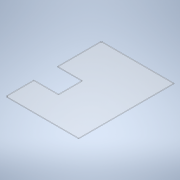
# Autodesk Inventor part: MountingWallSide2
Saved by Autodesk Inventor 2020 (Build 240168000, 168)
## iProperties
Created: 2020-04-26
Part Number: MountingWallSide2
Material: Типовые
Document SubType Name: Modeling
Designer: Михаил
Density: 1 g/cm^3
Appearance: По умолчанию
Author: Михаил
Autodesk Inventor part; units mm, degrees
ref_plane "YZ Plane" through (0, 0, 0) normal (1, 0, 0) x (0, 1, 0)
ref_plane "XZ Plane" through (0, 0, 0) normal (0, 1, 0) x (-1, 0, 0)
ref_plane "XY Plane" through (0, 0, 0) normal (0, 0, 1) x (1, 0, 0)
sketch "Эскиз1" plane through (0, 0, 0) normal (0, 1, 0) x (-1, 0, 0)
  line L0 (0, 0) -> (388, 0)
  line L1 (388, 0) -> (388, -508)
  line L2 (388, -508) -> (0, -508)
  line L3 (0, -508) -> (0, 0)
  dimension "d0" = 388
  dimension "d1" = 508
  constraints: 8 end point, 2 parallel, 1 horizontal, 1 perpendicular
  measures "d0" distance of L1.end L2.end
  measures "d1" distance of L0.end L1.end
extrude "Выдавливание1" add sketch "Эскиз1" along normal blind 4
sketch "Эскиз2" plane through (0, 4, 0) normal (0, 1, 0) x (1, 0, 0)
  line L0 (-388, 508) -> (-388, 0) projected
  line L1 (-388, 149) -> (-257, 149)
  line L2 (-257, 149) -> (-257, 275)
  line L3 (-257, 275) -> (-388, 275)
  line L4 (-388, 275) -> (-388, 149)
  line L5 (0, 0) -> (-5, 0)
  line L6 (-388, 0) -> (0, 0) projected
  line L7 (-388, 0) -> (-384, 0)
  line L8 (-384, 0) -> (-384, 4)
  line L9 (-384, 4) -> (-388, 4)
  line L10 (-388, 4) -> (-388, 0)
  line L11 (0, 508) -> (-388, 508) projected
  line L12 (-388, 508) -> (-384, 508)
  line L13 (-384, 508) -> (-384, 504)
  line L14 (-384, 504) -> (-388, 504)
  line L15 (-388, 504) -> (-388, 508)
  point P0 (-388, 275)
  dimension "d4" = 126
  dimension "d5" = 131
  dimension "d13" = 149
  dimension "d14" = 4
  dimension "d15" = 4
  dimension "d16" = 4
  dimension "d17" = 4
  constraints: 26 end point, 6 parallel, 4 horizontal, 3 perpendicular, 1 point on line
  measures "d4" distance of L1.end L2.end
  measures "d5" distance of L2.end L3.end
  measures "d13" distance between parallel lines of L6 L1
  measures "d14" distance of L9.end L8.end
  measures "d15" distance of L8.end L7.end
  measures "d16" distance of L13.end L14.end
  measures "d17" distance of L12.end L13.end
extrude "Выдавливание3" cut sketch "Эскиз2" against normal blind 10
